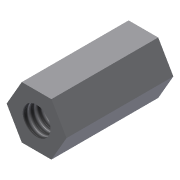
# Autodesk Inventor part: #8 .5 Hex Standoff
Saved by Autodesk Inventor 2014 (Build 180170000, 170)
## iProperties
Created: 2014-07-18
Part Number: #8 .5 Hex Standoff
Material: Generic
Document SubType Name: Modeling
Designer: Owner
Density: 1 g/cm^3
Appearance: Default
Author: Owner
Autodesk Inventor part; units mm, degrees
ref_plane "YZ Plane" through (0, 0, 0) normal (1, 0, 0) x (0, 1, 0)
ref_plane "XZ Plane" through (0, 0, 0) normal (0, 1, 0) x (-1, 0, 0)
ref_plane "XY Plane" through (0, 0, 0) normal (0, 0, 1) x (1, 0, 0)
sketch "Sketch1" plane through (0, 0, 0) normal (0, 0, 1) x (1, 0, 0)
  line L0 (-3.556, 0) -> (3.556, 0) construction
  line L1 (0, 3.1115) -> (0, -3.1115) construction
  line L2 (3.556, 0) -> (1.7596, 3.1115)
  line L3 (3.556, 0) -> (6.0601, 0) construction
  line L4 (-1.7596, -3.1115) -> (1.7596, -3.1115)
  line L5 (-3.556, 0) -> (-1.7596, 3.1115)
  line L6 (-3.556, 0) -> (-1.016, 0) construction
  line L7 (-3.556, 0) -> (-1.7596, -3.1115)
  line L8 (3.556, 0) -> (1.7596, -3.1115)
  line L9 (3.556, 0) -> (6.096, 0) construction
  line L10 (-1.7596, 3.1115) -> (1.7596, 3.1115)
  point P0 (0, 0)
  point P1 (0, 0)
  dimension "d0" = 7.112
  dimension "d2" = 6.223
  dimension "d4" = 120
  dimension "d7" = 60
  dimension "d9" = 120
  dimension "d10" = 2.5041
  dimension "d11" = 2.54
  dimension "d12" = 2.54
  constraints: 22 end point, 4 horizontal, 4 midpoint, 3 parallel, 1 coincident, 1 perpendicular
  measures "d0" distance of L0.start L0.end
  measures "d2" distance of L1.end L1.start
  measures "d4" angle of L3 L2
  measures "d7" angle of L6 L5
  measures "d9" angle of L8 L9
  measures "d10" distance of L0.end L3.end
  measures "d11" distance of L0.start L6.end
  measures "d12" distance of L0.end L9.end
extrude "Extrusion1" add sketch "Sketch1" against normal blind 12.7
ref_plane "Work Plane1" through (0, 0, 0) normal (0, 0, 1) x (1, 0, 0)
hole "Hole1" at (0, 0, 0) direction (0, 0, -1) diameter 3.302 end through all thread size "8-32 UNC" class "2B" standard "ANSI Unified Screw Threads"
body "Solid1"
